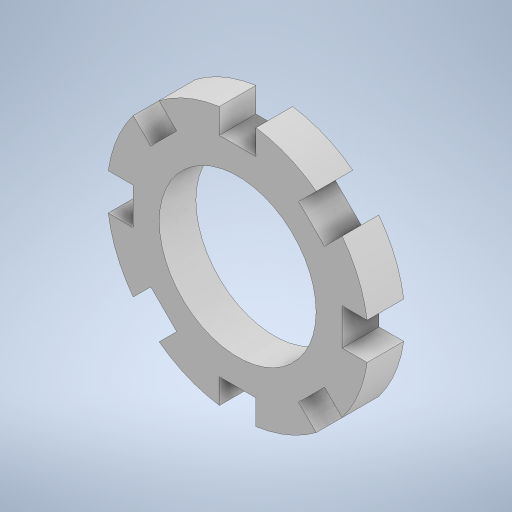
# Autodesk Inventor part: Vrhnji obrok
Saved by Autodesk Inventor 2023 (Build 270158000, 158)
## iProperties
Created: 2022-12-16
Part Number: Vrhnji obrok
Material: Generic
Document SubType Name: Modeling
Designer: David Zindović
Density: 1 g/cm^3
Appearance: Default
Author: David Zindović
Autodesk Inventor part; units mm, degrees
ref_plane "YZ Plane" through (0, 0, 0) normal (1, 0, 0) x (0, 1, 0)
ref_plane "XZ Plane" through (0, 0, 0) normal (0, 1, 0) x (-1, 0, 0)
ref_plane "XY Plane" through (0, 0, 0) normal (0, 0, 1) x (1, 0, 0)
sketch "Sketch1" plane through (0, 0, 0) normal (0, 0, 1) x (1, 0, 0)
  circle A0 centre (0, 0) radius 10
  circle A1 centre (0, 0) radius 12.5
  circle A2 centre (0, 0) radius 7.5
  line L0 (10, 0) -> (12.5, 0)
  line L1 (12.5, 0) -> (12.5, 1.75)
  line L2 (12.5, 1.75) -> (10, 1.75)
  line L3 (10, 1.75) -> (10, 0)
  line L4 (12.5, 0) -> (12.5, -1.75)
  line L5 (12.5, -1.75) -> (10, -1.75)
  line L6 (10, -1.75) -> (10, 0)
  line L7 (10.0763, 7.6014) -> (8.3085, 5.8336)
  line L8 (8.3085, 5.8336) -> (7.0711, 7.0711)
  line L9 (5.8336, 8.3085) -> (7.0711, 7.0711)
  line L10 (7.6014, 10.0763) -> (5.8336, 8.3085)
  line L11 (8.8388, 8.8388) -> (7.6014, 10.0763)
  line L12 (8.8388, 8.8388) -> (10.0763, 7.6014)
  line L13 (1.75, 12.5) -> (1.75, 10)
  line L14 (1.75, 10) -> (0, 10)
  line L15 (-1.75, 10) -> (0, 10)
  line L16 (-1.75, 12.5) -> (-1.75, 10)
  line L17 (0, 12.5) -> (-1.75, 12.5)
  line L18 (0, 12.5) -> (1.75, 12.5)
  line L19 (-7.6014, 10.0763) -> (-5.8336, 8.3085)
  line L20 (-5.8336, 8.3085) -> (-7.0711, 7.0711)
  line L21 (-8.3085, 5.8336) -> (-7.0711, 7.0711)
  line L22 (-10.0763, 7.6014) -> (-8.3085, 5.8336)
  line L23 (-8.8388, 8.8388) -> (-10.0763, 7.6014)
  line L24 (-8.8388, 8.8388) -> (-7.6014, 10.0763)
  line L25 (-12.5, 1.75) -> (-10, 1.75)
  line L26 (-10, 1.75) -> (-10, 0)
  line L27 (-10, -1.75) -> (-10, 0)
  line L28 (-12.5, -1.75) -> (-10, -1.75)
  line L29 (-12.5, 0) -> (-12.5, -1.75)
  line L30 (-12.5, 0) -> (-12.5, 1.75)
  line L31 (-10.0763, -7.6014) -> (-8.3085, -5.8336)
  line L32 (-8.3085, -5.8336) -> (-7.0711, -7.0711)
  line L33 (-5.8336, -8.3085) -> (-7.0711, -7.0711)
  line L34 (-7.6014, -10.0763) -> (-5.8336, -8.3085)
  line L35 (-8.8388, -8.8388) -> (-7.6014, -10.0763)
  line L36 (-8.8388, -8.8388) -> (-10.0763, -7.6014)
  line L37 (-1.75, -12.5) -> (-1.75, -10)
  line L38 (-1.75, -10) -> (0, -10)
  line L39 (1.75, -10) -> (0, -10)
  line L40 (1.75, -12.5) -> (1.75, -10)
  line L41 (0, -12.5) -> (1.75, -12.5)
  line L42 (0, -12.5) -> (-1.75, -12.5)
  line L43 (7.6014, -10.0763) -> (5.8336, -8.3085)
  line L44 (5.8336, -8.3085) -> (7.0711, -7.0711)
  line L45 (8.3085, -5.8336) -> (7.0711, -7.0711)
  line L46 (10.0763, -7.6014) -> (8.3085, -5.8336)
  line L47 (8.8388, -8.8388) -> (10.0763, -7.6014)
  line L48 (8.8388, -8.8388) -> (7.6014, -10.0763)
  point P0 (-1.75, 12.3769)
  point P1 (-7.5143, 9.9892)
  point P2 (-9.9892, 7.5143)
  point P3 (-12.3769, 1.75)
  point P4 (-12.3769, -1.75)
  point P5 (-9.9892, -7.5143)
  point P6 (-7.5143, -9.9892)
  point P7 (-1.75, -12.3769)
  point P8 (1.75, -12.3769)
  point P9 (7.5143, -9.9892)
  point P10 (9.9892, -7.5143)
  point P11 (12.3769, -1.75)
  point P12 (12.3769, 1.75)
  point P13 (9.9892, 7.5143)
  point P14 (7.5143, 9.9892)
  point P15 (1.75, 12.3769)
  dimension "d10" = 20
  dimension "d11" = 2.5
  dimension "d12" = 2.5
  dimension "d13" = 1.75
  dimension "d16" = 360
  constraints: 98 end point, 2 centre point, 2 parallel, 2 symmetric about line, 1 coincident, 1 horizontal, 1 horizontal alignment, 1 perpendicular, 99 other
  measures "d13" distance of L2.end L0.start
extrude "Extrusion1" add sketch "Sketch1" along normal mid plane 3.5 contours A0 | L6 L5 A1 L46 L45 A0 | A0 L8 L7 A1 L2 L3 | A0 L14 L13 A1 L10 L9 | L44 L43 A1 L40 L39 A0 | A0 L20 L19 A1 L16 L15 | L38 L37 A1 L34 L33 A0 | A0 L26 L25 A1 L22 L21 | L32 L31 A1 L28 L27 A0
body "Solid1"
